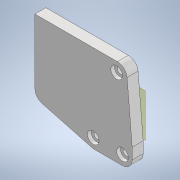
# Autodesk Inventor part: BOWDEN MOUNT
Saved by Autodesk Inventor 2020 (Build 240168000, 168)
## iProperties
Created: 2019-06-20
Part Number: BOWDEN MOUNT
Material: Generic
Document SubType Name: Modeling
Designer: pepd9
Density: 1 g/cm^3
Appearance: Default
Author: pepd9
Autodesk Inventor part; units mm, degrees
ref_plane "YZ Plane" through (0, 0, 0) normal (1, 0, 0) x (0, 1, 0)
ref_plane "XZ Plane" through (0, 0, 0) normal (0, 1, 0) x (-1, 0, 0)
ref_plane "XY Plane" through (0, 0, 0) normal (0, 0, 1) x (1, 0, 0)
ref_plane "Work Plane2" through (0, 0, 0) normal (0, 0, 1) x (1, 0, 0)
sketch "Sketch1" plane through (0, 0, 0) normal (0, 0, 1) x (1, 0, 0)
  line L0 (-10, 22.5) -> (10, 22.5)
  line L1 (10, 22.5) -> (10, -22.5)
  line L2 (10, -22.5) -> (-10, -22.5)
  line L3 (-10, -22.5) -> (-10, 22.5)
  circle A0 centre (0, 17.5) radius 1.25
  circle A1 centre (5, -17.5) radius 1.25
  point P0 (0, 0)
  dimension "d38" = 20
  dimension "d39" = 45
  dimension "d40" = 2.5
  dimension "d41" = 2.5
  dimension "d42" = 10
  dimension "d43" = 5
  dimension "d44" = 5
  dimension "d45" = 5
  constraints: 8 end point, 2 centre point, 2 parallel, 1 horizontal, 1 perpendicular
  measures "d38" distance of L0.start L0.end
  measures "d39" distance of L2.end L0.start
  measures "d40" diameter of A0
  measures "d41" diameter of A1
  measures "d42" distance from line of L1 A0.centre
  measures "d43" distance from line of L0 A0.centre
  measures "d44" distance from line of L2 A1.centre
  measures "d45" distance from line of L1 A1.centre
extrude "Extrusion1" add sketch "Sketch1" along normal blind 3.65 contours L0 L1 L2 L3 | A0 | A1
sketch "Sketch2" plane through (-10, 118.2358, 3.65) normal (-1, 0, 0) x (0, 0, 1)
  line L0 (-3.65, -95.7358) -> (-3.65, -140.7358) projected
  line L1 (-3.65, -140.7358) -> (0, -140.7358) projected
  line L2 (0, -95.7358) -> (0, -140.7358) projected
  line L3 (-3.65, -95.7358) -> (0, -95.7358) projected
  point P0 (-3.65, -118.2358)
extrude "Extrusion2" add sketch "Sketch2" along normal blind 30
sketch "Sketch3" plane through (0, 0, 3.65) normal (0, 0, 1) x (1, 0, 0)
  line L0 (10, -22.5) -> (10, 22.5) projected
  line L1 (10, 22.5) -> (-40, 22.5) projected
  line L2 (-40, -22.5) -> (-40, 22.5) projected
  line L3 (10, -22.5) -> (-40, -22.5) projected
  circle A0 centre (0, 17.5) radius 3 construction
  circle A1 centre (5, -17.5) radius 3 construction
  point P0 (0, 0)
  dimension "d48" = 6
  dimension "d49" = 6
  constraints: 2 centre point
  measures "d48" diameter of A0
  measures "d49" diameter of A1
extrude "Extrusion3" add sketch "Sketch3" along normal blind 2
ref_plane "Work Plane3" through (0, 0, 0) normal (0, 0, -1) x (-1, 0, 0)
sketch "Sketch10" plane through (0, 0, 5.65) normal (0, 0, 1) x (1, 0, 0)
  circle A0 centre (-10, -17.5) radius 2.5953
  line L0 (-40, -22.5) -> (10, -22.5) projected
  line L1 (10, -22.5) -> (10, 22.5) projected
  circle A1 centre (5, -17.5) radius 2.5953
  circle A2 centre (2, 17.5) radius 2.5953
  line L2 (10, 22.5) -> (-40, 22.5) projected
  point P0 (0, 0)
  dimension "d75" = 5
  dimension "d76" = 20
  dimension "d77" = 8
  dimension "d78" = 5
  dimension "d79" = 5
  dimension "d80" = 5
  constraints: 3 centre point
  measures "d75" distance from line of L0 A0.centre
  measures "d76" distance from line of L1 A0.centre
  measures "d77" distance from line of L1 A2.centre
  measures "d78" distance from line of L2 A2.centre
  measures "d79" distance from line of L1 A1.centre
  measures "d80" distance from line of A1.centre L0
hole "Hole4" at (-10, -17.5, 5.65) at (5, -17.5, 5.65) at (2, 17.5, 5.65) direction (0, 0, -1) diameter 3.1 end through all counterbore diameter 6 counterbore depth 1.9
sketch "Sketch11" plane through (0, 0, 5.65) normal (0, 0, 1) x (1, 0, 0)
  circle A0 centre (5, -17.5) radius 3 projected
  circle A1 centre (-10, -17.5) radius 3 projected
  circle A2 centre (2, 17.5) radius 3 projected
  line L0 (-40, -22.5) -> (10, -22.5) projected
  line L1 (10, -22.5) -> (10, 22.5) projected
  line L2 (10, 22.5) -> (-40, 22.5) projected
  line L3 (-40, 22.5) -> (-40, -22.5) projected
  line L4 (-40, -22.5) -> (10, -22.5) projected
  line L5 (-10.1436, -22.5) -> (-40, -14.5)
  line L6 (10, 22.5) -> (-40, 22.5) projected
  line L7 (7, 22.5) -> (10, -11.7902)
  point P0 (0, 0)
  dimension "d81" = 15
  dimension "d82" = 8
  dimension "d83" = 5
  dimension "d84" = 3
  constraints: 4 end point, 4 point on line
  measures "d81" angle of L0 L5
  measures "d82" distance from line of L5.end L0
  measures "d83" angle of L1 L7
  measures "d84" distance from line of L1 L7.start
extrude "Extrusion7" cut sketch "Sketch11" against normal through all contours L3 L5 L0 | L7 L2 L1
fillet "Fillet1" radius 5 3 edges at (10, -22.5, 2.825) (7, 22.5, 2.825) (-40, -14.5, 2.825)
sketch "Sketch12" plane through (0, 0, 5.65) normal (0, 0, 1) x (1, 0, 0)
  arc A0 (-24.0463, 1.5877) -> (-17.4606, 8.5418) centre (-23.3781, 7.5504) ccw
  arc A1 (-17.4606, 8.5418) -> (-23.6797, 15.6342) centre (-24.4593, 8.6778) ccw
  arc A2 (-30.4648, 16.3946) -> (-32.024, 2.4817) centre (-32.4095, 9.5688) ccw
  line L0 (-32.024, 2.4817) -> (-24.0463, 1.5877)
  line L1 (-23.6797, 15.6342) -> (-30.4648, 16.3946)
  point P0 (0, 0)
  constraints: 6 point on circle, 4 end point, 3 centre point, 13 other
extrude "Extrusion8" cut sketch "Sketch12" against normal through all
sketch "Sketch13" plane through (0, 0, 0) normal (0, 0, -1) x (-1, 0, 0)
  arc A0 (32.024, 2.4817) -> (30.4648, 16.3946) centre (32.4095, 9.5688) ccw projected
  line L0 (32.024, 2.4817) -> (24.0463, 1.5877) projected
  arc A1 (17.4606, 8.5418) -> (24.0463, 1.5877) centre (23.3781, 7.5504) ccw projected
  arc A2 (23.6797, 15.6342) -> (17.4606, 8.5418) centre (24.4593, 8.6778) ccw projected
  line L1 (23.6797, 15.6342) -> (30.4648, 16.3946) projected
  arc A3 (36.2941, -15.493) -> (40, -10.6634) centre (35, -10.6634) ccw projected
  line L2 (40, 22.5) -> (40, -10.6634) projected
  line L3 (-2.4183, 22.5) -> (40, 22.5) projected
  arc A4 (-2.4183, 22.5) -> (-7.3993, 17.9358) centre (-2.4183, 17.5) ccw projected
  line L4 (-7.3993, 17.9358) -> (-10, -11.7902) projected
  line L5 (-10, -17.5) -> (-10, -11.7902) projected
  arc A5 (-10, -17.5) -> (-5, -22.5) centre (-5, -17.5) ccw projected
  line L6 (-5, -22.5) -> (10.1436, -22.5) projected
  line L7 (10.1436, -22.5) -> (36.2941, -15.493) projected
  circle A6 centre (-5, -17.5) radius 1.55 projected
  circle A7 centre (10, -17.5) radius 1.55 projected
  circle A8 centre (-2, 17.5) radius 1.55 projected
  line L8 (2.3679, 22.8864) -> (2.6218, 20.62)
  line L9 (2.3679, 22.8864) -> (5.0151, 26.2019)
  line L10 (40.1666, 30.1412) -> (5.0151, 26.2019)
  line L11 (40.1666, 30.1412) -> (43.482, 27.494)
  line L12 (43.482, 27.494) -> (47.2776, -6.3746)
  line L13 (47.2776, -6.3746) -> (44.6304, -9.69)
  line L14 (44.6304, -9.69) -> (34.1957, -10.8594)
  point P0 (0, 0)
  point P1 (2.4112, 22.5)
  point P2 (40, -10.2089)
  constraints: 14 end point, 15 other
extrude "Extrusion9" add sketch "Sketch13" against normal up to surface (5.65 mm away) contours L2 L3 L8 L9 L10 L11 L12 L13 L14
sketch "Sketch14" plane through (0, 0, 0) normal (0, 0, -1) x (-1, 0, 0)
  circle A0 centre (37.6266, 25.8315) radius 1.7
  circle A1 centre (9.4116, 22.6695) radius 1.7
  circle A2 centre (10.7819, -8.452) radius 2.205
  circle A3 centre (41.5891, -4.9995) radius 1.7
  point P0 (0, 0)
  constraints: 4 centre point, 8 other
hole "Hole5" at (-9.4116, 22.6695, 0) at (-37.6266, 25.8315, 0) at (-41.5891, -4.9995, 0) at (-10.7819, -8.452, 0) direction (0, 0, 1) diameter 3 end through all counterbore diameter 6 counterbore depth 2.5
body "Solid1"
